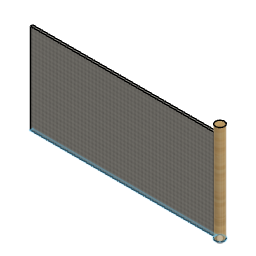
_2 per ext.cfb9fc78-3ace-48db-8203-243c851f6d8b (Autodesk Fusion 360 design; units mm, degrees)
Autodesk Fusion 360 part; units mm, degrees
sketch "sketch 329" plane through (0, 0, 0) normal (0, 0, 1) x (1, 0, 0)
  line L0 (704.8107, -77.7875) -> (704.8107, -74.6125)
  line L1 (704.8107, -74.6125) -> (445.4282, -74.6125)
  line L2 (445.4282, -74.6125) -> (445.4282, -77.7875)
  line L3 (445.4282, -77.7875) -> (704.8107, -77.7875)
  circle A0 centre (711.2, -76.2) radius 6.35
extrude "Extrude1" add sketch "sketch 329" along normal blind 127 makes body 1 at (531.8891, -77.7875, 42.3333) makes body 2 at (711.3583, -69.852, 84.6667)
extrude "Extrude2" add 1 faces at (712.9489, -74.3767, 127) along direction (0, 0, 1) blind 12.7 on bodies 2 bodies 2
